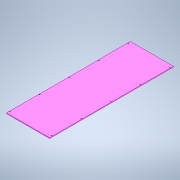
# Autodesk Inventor part: Base
Saved by Autodesk Inventor 2021 (Build 250183000, 183)
## iProperties
Created: 2022-02-04
Part Number: Base
Material: Generic
Document SubType Name: Modeling
Designer: tlar613
Density: 1 g/cm^3
Appearance: Default
Author: tlar613
Autodesk Inventor part; units mm, degrees
ref_plane "YZ Plane" through (0, 0, 0) normal (1, 0, 0) x (0, 1, 0)
ref_plane "XZ Plane" through (0, 0, 0) normal (0, 1, 0) x (-1, 0, 0)
ref_plane "XY Plane" through (0, 0, 0) normal (0, 0, 1) x (1, 0, 0)
sketch "Sketch1" plane through (0, 0, 0) normal (0, 1, 0) x (-1, 0, 0)
  line L0 (165, 474.1) -> (-165, 474.1)
  line L1 (-165, 474.1) -> (-165, -474.1)
  line L2 (-165, -474.1) -> (165, -474.1)
  line L3 (165, -474.1) -> (165, 474.1)
  line L4 (0, -663.74) -> (0, 663.74) projected
  line L5 (-231, 0) -> (231, 0) projected
  circle A0 centre (159, -452) radius 3
  circle A1 centre (159, -226) radius 3
  circle A2 centre (159, 0) radius 3
  circle A3 centre (159, 226) radius 3
  circle A4 centre (159, 452) radius 3
  circle A5 centre (-159, -452) radius 3
  circle A6 centre (-159, -226) radius 3
  circle A7 centre (-159, 0) radius 3
  circle A8 centre (-159, 226) radius 3
  circle A9 centre (-159, 452) radius 3
  point P0 (0, 0)
  point P1 (156, 0)
  point P2 (162, 0)
  point P3 (165, 0)
  point P4 (-165, 0)
  point P5 (-162, 0)
  point P6 (-156, 0)
  dimension "d0" = 948.2
  dimension "d1" = 330
  dimension "d4" = 6
  dimension "d5" = 6
  dimension "d6" = 6
  dimension "d7" = 6
  dimension "d8" = 6
  dimension "d9" = 6
  dimension "d10" = 6
  dimension "d11" = 6
  dimension "d12" = 6
  dimension "d13" = 6
  dimension "d14" = 6
  dimension "d15" = 22.1
  dimension "d16" = 22.1
  dimension "d17" = 226
  dimension "d19" = 226
  dimension "d20" = 226
  dimension "d21" = 226
  dimension "d22" = 226
  dimension "d23" = 226
  dimension "d24" = 226
  dimension "d25" = 226
  constraints: 10 centre point, 9 equal radius, 8 end point, 2 parallel, 1 horizontal, 1 perpendicular, 2 other
  measures "d0" distance of L2.end L0.start
  measures "d1" distance of L1.end L2.end
  measures "d4" diameter of A0
  measures "d5" distance from line of L3 A0.centre
  measures "d6" distance from line of L3 A1.centre
  measures "d7" distance from line of L3 A2.centre
  measures "d8" distance from line of L3 A3.centre
  measures "d9" distance from line of L3 A4.centre
  measures "d10" distance from line of L1 A9.centre
  measures "d11" distance from line of L1 A8.centre
  measures "d12" distance from line of L1 A7.centre
  measures "d13" distance from line of L1 A6.centre
  measures "d14" distance from line of L1 A5.centre
  measures "d15" distance from line of L2 A0.centre
  measures "d16" distance from line of L2 A5.centre
  measures "d17" distance of A1.centre A0.centre
  measures "d19" distance of A2.centre A1.centre
  measures "d20" distance of A3.centre A2.centre
  measures "d21" distance of A4.centre A3.centre
  measures "d22" distance of A6.centre A5.centre
  measures "d23" distance of A7.centre A6.centre
  measures "d24" distance of A8.centre A7.centre
  measures "d25" distance of A9.centre A8.centre
extrude "Extrusion1" add sketch "Sketch1" along normal blind 5 contours L3 L5 A2 L4 L0 | L4 L5 A7 L1 L0 | L3 L2 L4 L5 A2 | L4 L2 L1 L5 A7
body "Solid1"
